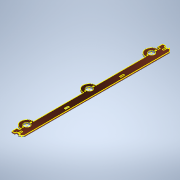
# Autodesk Inventor part: chassis_1_1
Saved by Autodesk Inventor 2022 (Build 260153000, 153)
## iProperties
Created: 2023-03-24
Part Number: chassis_1_1
Material: 一般
Document SubType Name: Modeling
Designer: Johnny Jou
Density: 1 g/cm^3
Appearance: 預設
Author: Johnny Jou
Autodesk Inventor part; units mm, degrees
ref_plane "YZ Plane" through (0, 0, 0) normal (1, 0, 0) x (0, 1, 0)
ref_plane "XZ Plane" through (0, 0, 0) normal (0, 1, 0) x (-1, 0, 0)
ref_plane "XY Plane" through (0, 0, 0) normal (0, 0, 1) x (1, 0, 0)
sketch "草圖1" plane through (0, 0, 0) normal (0, 1, 0) x (-1, 0, 0)
  line L0 (0, 0) -> (0, -306)
  arc A0 (15, -165.4599) -> (15, -140.5401) centre (16, -153) ccw
  circle A1 centre (16, -153) radius 26 construction
  line L1 (15, -296) -> (15, -165.4599)
  line L2 (15, -140.5401) -> (15, -10)
  circle A2 centre (16, -144.5) radius 1
  circle A3 centre (16, -161.5) radius 1
  line L3 (20, 0) -> (20, -10)
  line L4 (20, -10) -> (15, -10)
  line L5 (0, -10) -> (0, 0)
  line L6 (6, 0) -> (6, -3)
  line L7 (6, -3) -> (14, -3)
  line L8 (14, -3) -> (14, 0)
  line L9 (0, 0) -> (6, 0)
  line L10 (14, 0) -> (20, 0)
  line L11 (15, 0) -> (14, 0)
  line L12 (6, 0) -> (0, 0)
  line L13 (20, -306) -> (20, -296)
  line L14 (20, -296) -> (15, -296)
  line L15 (0, -290) -> (0, -306)
  line L16 (6, -306) -> (6, -303)
  line L17 (6, -303) -> (14, -303)
  line L18 (14, -303) -> (14, -306)
  line L19 (0, -306) -> (6, -306)
  line L20 (14, -306) -> (20, -306)
  dimension "d1" = 15
  dimension "d2" = 25
  dimension "d3" = 52
  dimension "d4" = 16
  dimension "d6" = 2
  dimension "d7" = 17
  dimension "d8" = 8.5
  dimension "d9" = 10
  dimension "d10" = 20
  dimension "d11" = 8
  dimension "d12" = 3
  dimension "d13" = 6
  dimension "d15" = 3
  dimension "d16" = 8
  dimension "d17" = 6
  dimension "d34" = 306
  dimension "d35" = 153
  dimension "d36" = 10
  dimension "d55" = 8.5
  dimension "d56" = 15
  dimension "d57" = 15
  constraints: 42 end point, 10 parallel, 6 horizontal, 6 perpendicular, 4 centre point, 2 coincident, 2 collinear, 2 point on circle, 1 equal radius, 1 vertical alignment
  measures "d1" distance of L11.start L0.start
  measures "d2" diameter of A0
  measures "d3" diameter of A1
  measures "d4" distance from line of L0 A0.centre
  measures "d6" diameter of A2
  measures "d7" distance of A3.centre A2.centre
  measures "d8" distance of A0.centre A3.centre
  measures "d9" distance of L3.start L3.end
  measures "d10" distance between parallel lines of L0 L3
  measures "d11" distance of L6.end L7.end
  measures "d12" distance of L7.end L8.end
  measures "d13" distance between parallel lines of L5 L6
  measures "d15" distance of L17.end L18.end
  measures "d16" distance of L16.end L17.end
  measures "d17" distance between parallel lines of L0 L16
  measures "d34" distance of L0.start L0.end
  measures "d35" distance from line of L19 A0.centre
  measures "d36" distance of L13.start L13.end
  measures "d55" distance of A0.centre A2.centre
  measures "d56" distance between parallel lines of L0 L1
  measures "d57" distance between parallel lines of L0 L2
extrude "擠出1" add sketch "草圖1" along normal blind 3
sketch "草圖2" plane through (0, 3, 0) normal (0, 1, 0) x (1, 0, 0)
  line L0 (-7, 205) -> (-4, 205)
  line L1 (-4, 205) -> (-4, 213)
  line L2 (-4, 213) -> (-7, 213)
  line L3 (-7, 213) -> (-7, 205)
  arc A0 (-15, 165.4599) -> (-15, 140.5401) centre (-16, 153) ccw projected
  line L4 (-15, 140.5401) -> (-15, 10) projected
  circle A1 centre (-16, 153) radius 12.5 construction
  line L5 (0, 0) -> (0, 306) projected
  line L6 (-11, 4) -> (-8, 4)
  line L7 (-8, 4) -> (-8, 10)
  line L8 (-8, 10) -> (-11, 10)
  line L9 (-11, 10) -> (-11, 4)
  line L10 (-14, 3) -> (-6, 3) projected
  line L11 (-11, 296) -> (-8, 296)
  line L12 (-8, 296) -> (-8, 302)
  line L13 (-8, 302) -> (-11, 302)
  line L14 (-11, 302) -> (-11, 296)
  line L15 (-6, 303) -> (-14, 303) projected
  line L16 (-7, 93) -> (-4, 93)
  line L17 (-4, 93) -> (-4, 101)
  line L18 (-4, 101) -> (-7, 101)
  line L19 (-7, 101) -> (-7, 93)
  line L20 (-15, 296) -> (-15, 165.4599) projected
  dimension "d20" = 8
  dimension "d21" = 3
  dimension "d22" = 60
  dimension "d23" = 4
  dimension "d24" = 6
  dimension "d25" = 3
  dimension "d27" = 1
  dimension "d28" = 6
  dimension "d29" = 3
  dimension "d31" = 1
  dimension "d58" = 3
  dimension "d59" = 8
  dimension "d60" = 60
  dimension "d69" = 4
  dimension "d70" = 4
  constraints: 32 end point, 8 parallel, 4 horizontal, 4 perpendicular, 1 coincident, 1 collinear, 3 other
  measures "d20" distance of L2.end L0.start
  measures "d21" distance of L1.end L2.end
  measures "d22" distance from line of A0.centre L2
  measures "d23" distance between parallel lines of L5 L1
  measures "d24" distance of L8.end L6.start
  measures "d25" distance of L7.end L8.end
  measures "d27" distance between parallel lines of L10 L6
  measures "d28" distance of L13.end L11.start
  measures "d29" distance of L11.start L11.end
  measures "d31" distance between parallel lines of L15 L13
  measures "d58" distance of L17.end L18.end
  measures "d59" distance of L16.end L17.end
  measures "d60" distance from line of A0.centre L16
  measures "d69" distance between parallel lines of L20 L14
  measures "d70" distance between parallel lines of L4 L9
extrude "擠出2" cut sketch "草圖2" against normal up to surface (3 mm away)
sketch "草圖3" plane through (0, 3, 0) normal (0, 1, 0) x (1, 0, 0)
  arc A0 (-15, 165.4599) -> (-15, 140.5401) centre (-16, 153) ccw projected
  circle A1 centre (-16, 153) radius 6
  point P0 (0, 0)
  dimension "d37" = 12
  constraints: 1 centre point, 1 coincident
  measures "d37" diameter of A1
extrude "擠出3" cut sketch "草圖3" against normal up to surface (3 mm away)
sketch "草圖4" plane through (0, 3, 0) normal (0, 1, 0) x (1, 0, 0)
  circle A0 centre (-16, 153) radius 6 projected
  arc A1 (-15, 165.4599) -> (-15, 140.5401) centre (-16, 153) ccw projected
  circle A2 centre (-16, 144.5) radius 1 projected
  circle A3 centre (-16, 161.5) radius 1 projected
  circle A4 centre (-16, 26.5) radius 12.5
  circle A5 centre (-16, 26.5) radius 6
  circle A6 centre (-16, 35) radius 1
  circle A7 centre (-16, 18) radius 1
  line L0 (-15, 140.5401) -> (-15, 10) projected
  circle A8 centre (-16, 279.5) radius 12.5
  circle A9 centre (-16, 279.5) radius 6
  circle A10 centre (-16, 288) radius 1
  circle A11 centre (-16, 271) radius 1
  point P0 (0, 0)
  point P1 (-15, 14.0401)
  point P2 (-15, 38.9599)
  dimension "d40" = 2
  dimension "d41" = 12
  dimension "d42" = 25
  dimension "d43" = 17
  dimension "d44" = 8.5
  dimension "d45" = 126.5
  dimension "d48" = 253
  constraints: 8 centre point, 3 vertical alignment, 2 coincident, 1 equal radius, 1 vertical, 8 other
  measures "d40" diameter of A6
  measures "d41" diameter of A5
  measures "d42" diameter of A4
  measures "d43" distance of A7.centre A6.centre
  measures "d44" distance of A4.centre A6.centre
  measures "d45" distance of A0.centre A4.centre
  measures "d48" distance of A4.centre A8.centre
extrude "擠出4" add sketch "草圖4" against normal up to surface (3 mm away) contours A4 L0 A5 | L0 A5 A4 | A8
sketch "草圖6" plane through (0, 3, 0) normal (0, 1, 0) x (1, 0, 0)
  arc A0 (-15, 32.4161) -> (-15, 20.5839) centre (-16, 26.5) ccw projected
  arc A1 (-15, 285.4161) -> (-15, 273.5839) centre (-16, 279.5) ccw projected
  line L0 (-15, 285.4161) -> (-15, 273.5839) projected
  circle A2 centre (-16, 279.5) radius 6
  line L1 (-15, 32.4161) -> (-15, 20.5839) projected
  circle A3 centre (-16, 26.5) radius 6
  point P0 (0, 0)
  point P1 (-15, 273.5839)
  point P2 (-15, 32.4161)
  constraints: 2 coincident, 6 other
extrude "擠出" cut sketch "草圖6" against normal up to surface (3 mm away) contours A3 L1 | L0 A1 | A2 L0
chamfer "倒角1" distance 6 angle 45 1 edges at (0, 1.5, -306)
chamfer "倒角2" distance 6 angle 45 1 edges at (0, 1.5, 0)
sketch "草圖7" plane through (0, 3, 0) normal (0, 1, 0) x (1, 0, 0)
  circle A0 centre (-16, 279.5) radius 6 projected
  circle A1 centre (-16, 26.5) radius 6 projected
  circle A2 centre (-16, 271) radius 1 projected
  line L0 (0, 6) -> (-6, 0) projected
  line L1 (0, 6) -> (0, 300) projected
  line L2 (-6, 306) -> (0, 300) projected
  line L3 (-6, 306) -> (-6, 303) projected
  line L4 (-6, 303) -> (-14, 303) projected
  line L5 (-14, 303) -> (-14, 306) projected
  line L6 (-14, 306) -> (-20, 306) projected
  line L7 (-20, 306) -> (-20, 296) projected
  line L8 (-20, 296) -> (-15, 296) projected
  line L9 (-15, 296) -> (-15, 291.9599) projected
  arc A3 (-15, 291.9599) -> (-15, 267.0401) centre (-16, 279.5) ccw projected
  line L10 (-15, 267.0401) -> (-15, 165.4599) projected
  arc A4 (-15, 165.4599) -> (-15, 140.5401) centre (-16, 153) ccw projected
  line L11 (-15, 140.5401) -> (-15, 38.9599) projected
  arc A5 (-15, 38.9599) -> (-15, 14.0401) centre (-16, 26.5) ccw projected
  line L12 (-15, 14.0401) -> (-15, 10) projected
  line L13 (-15, 10) -> (-20, 10) projected
  line L14 (-20, 10) -> (-20, 0) projected
  line L15 (-20, 0) -> (-14, 0) projected
  line L16 (-14, 0) -> (-14, 3) projected
  line L17 (-14, 3) -> (-6, 3) projected
  line L18 (-6, 3) -> (-6, 0) projected
  circle A6 centre (-16, 35) radius 1 projected
  circle A7 centre (-16, 288) radius 1 projected
  circle A8 centre (-16, 161.5) radius 1 projected
  circle A9 centre (-16, 144.5) radius 1 projected
  line L19 (-8, 4) -> (-11, 4) projected
  line L20 (-11, 4) -> (-11, 10) projected
  line L21 (-11, 10) -> (-8, 10) projected
  line L22 (-8, 10) -> (-8, 4) projected
  line L23 (-8, 302) -> (-8, 296) projected
  line L24 (-8, 296) -> (-11, 296) projected
  line L25 (-11, 296) -> (-11, 302) projected
  line L26 (-11, 302) -> (-8, 302) projected
  line L27 (-4, 93) -> (-7, 93) projected
  line L28 (-7, 93) -> (-7, 101) projected
  line L29 (-7, 101) -> (-4, 101) projected
  line L30 (-4, 101) -> (-4, 93) projected
  line L31 (-4, 213) -> (-4, 205) projected
  line L32 (-4, 205) -> (-7, 205) projected
  line L33 (-7, 205) -> (-7, 213) projected
  line L34 (-7, 213) -> (-4, 213) projected
  circle A10 centre (-16, 153) radius 6 projected
  circle A11 centre (-16, 18) radius 1 projected
  point P0 (0, 0)
equation "\"d8\" = 0.5 * d7"
equation "\"d31\" = d27"
equation "\"d58\" = d21"
equation "\"d59\" = d20"
equation "\"d60\" = d22"
equation "\"d44\" = 0.5 * d43"
equation "\"d48\" = 2 * d45"
